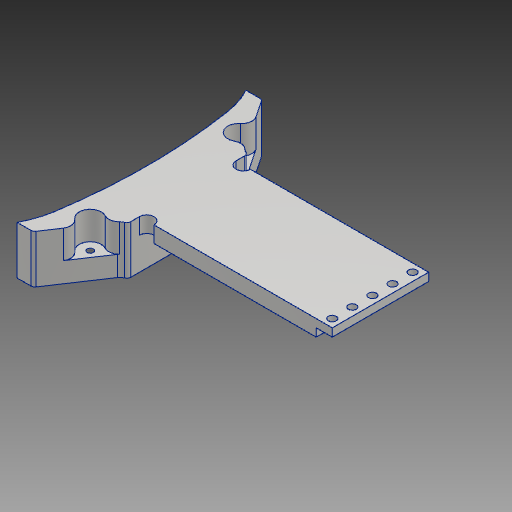
# Autodesk Inventor part: Kicker Sichel
Saved by Autodesk Inventor 2019.4 (Build 234330000, 330)
## iProperties
Part Number: Kicker Sichel
Material: Aluminium 6061
Document SubType Name: Modeling
Designer: rYan
Mass: 26.3222 g
Surface Area: 53.2988 cm^2
Volume: 9.74896 cm^3
Density: 2.7 g/cm^3
Appearance: Aluminium - flach
Author: rYan
Autodesk Inventor part; units mm, degrees
ref_plane "YZ Plane" through (0, 0, 0) normal (1, 0, 0) x (0, 1, 0)
ref_plane "XZ Plane" through (0, 0, 0) normal (0, 1, 0) x (-1, 0, 0)
ref_plane "XY Plane" through (0, 0, 0) normal (0, 0, 1) x (1, 0, 0)
sketch "Skizze1" plane through (0, 0, 0) normal (0, 0, 1) x (1, 0, 0)
  line L0 (3.6, 12) -> (48, 12)
  line L1 (48, 12) -> (48, -12)
  line L2 (48, -12) -> (3.6, -12)
  line L3 (-189.6, 0) -> (87.6, 0) projected
  line L4 (-1, 15) -> (-10, 28.5)
  line L5 (-1, -15) -> (-10, -28.5)
  line L6 (-10, -28.5) -> (-14, -28.5)
  line L7 (-10, 28.5) -> (-14, 28.5)
  arc A0 (-11.6616, 21.5053) -> (-14, 28.5) centre (-33.4005, 18.1259) ccw
  arc A1 (-14, -28.5) -> (-11.6616, -21.5053) centre (-33.4005, -18.1259) ccw
  arc A2 (-11.6616, -21.5053) -> (-11.6616, 21.5053) centre (-150, 0) ccw
  line L8 (-10, 28.5) -> (-10, -28.5) construction
  line L9 (0, 40.0382) -> (0, -40.0382) projected
  line L10 (-2, 12.5) -> (-2, -9.8115) construction
  arc A3 (0, 12) -> (3.6, 12) centre (1.8, 12) ccw
  arc A4 (3.6, -12) -> (0, -12) centre (1.8, -12) ccw
  line L11 (0, 12) -> (0, 15)
  line L12 (0, 15) -> (-1, 15)
  line L13 (0, -12) -> (0, -15)
  line L14 (0, -15) -> (-1, -15)
  point P0 (0, 0)
  dimension "d2" = 24
  dimension "d51" = 22
  dimension "d52" = 140
  dimension "d54" = 4
  dimension "d55" = 57
  dimension "d59" = 8
  dimension "d60" = 2
  dimension "d64" = 0
  dimension "d73" = 1.8
  dimension "d75" = 48
  dimension "d76" = 30
  dimension "d77" = 1
  constraints: 26 end point, 10 point on circle, 7 point on line, 5 centre point, 4 perpendicular, 3 horizontal, 3 tangent, 3 vertical, 1 parallel, 7 other
  measures "d2" distance of L0.end L1.end
  measures "d51" radius of A0
  measures "d52" radius of A2
  measures "d54" distance from line of L7.end L8
  measures "d55" distance between parallel lines of L6 L7
  measures "d59" distance between parallel lines of L10 L8
  measures "d60" distance between parallel lines of L9 L10
  measures "d64" distance from line of L8 L4.end
  measures "d73" radius of A3
  measures "d75" distance between parallel lines of L1 L9
  measures "d76" distance between parallel lines of L14 L12
  measures "d77" distance of L11.end L4.start
extrude "Extrusion1" add sketch "Skizze1" along normal blind 12
sketch "Skizze8" plane through (0, 0, 12) normal (0, 0, 1) x (1, 0, 0)
  line L0 (-189.6, 0) -> (87.6, 0) projected
  arc A0 (-11.6616, -21.5053) -> (-11.6616, 21.5053) centre (-150, 0) ccw projected
  line L1 (-1, 15) -> (-10, 28.5) projected
  line L2 (-11.2277, 18.5) -> (-3.3333, 18.5) construction
  point P0 (0, 0)
  point P1 (-5.7805, 18.5)
  point P2 (-5.7805, -18.5)
  point P3 (-7.2805, 18.5)
  dimension "d65" = 18.5
  dimension "d80" = 1.5
  constraints: 2 end point, 2 point on line, 1 horizontal, 1 midpoint, 1 point on circle, 1 symmetric about line
  measures "d65" distance between parallel lines of L0 L2
  measures "d80" distance of point (-7.281, 18.5) point (-5.781, 18.5)
hole "Bohrung4" at (-5.7805, 18.5, 12) at (-5.7805, -18.5, 12) direction (0, 0, -1) diameter 1.567 end through all counterbore diameter 5.5 counterbore depth 7 thread size "M2x0.4" class "6H" standard "ISO Metric profile"
sketch "Skizze2" plane through (0, 0, 0) normal (0, 0, -1) x (-1, 0, 0)
  line L0 (-48, -12) -> (-3.6, -12) projected
  line L1 (-48, 12) -> (-48, -12) projected
  line L2 (-48, 12) -> (-3.6, 12) projected
  line L3 (0, -12) -> (-48, -12)
  line L4 (-48, -12) -> (-48, 12)
  line L5 (-48, 12) -> (0, 12)
  line L6 (-3.6, 12) -> (-48, 12) projected
  line L7 (0, 12) -> (0, -12)
  point P0 (0, 0)
  point P1 (0, -12.5)
  point P2 (0, 12.5)
  point P3 (-3.6, -12)
  constraints: 8 end point, 2 horizontal, 1 midpoint, 1 parallel, 1 perpendicular, 1 vertical, 4 other
extrude "Extrusion2" cut sketch "Skizze2" against normal blind 8
sketch "Skizze3" plane through (0, 0, 8) normal (0, 0, -1) x (-1, 0, 0)
  line L0 (-3.6, -12) -> (-48, -12) projected
  line L1 (-48, -12) -> (-48, 12) projected
  line L2 (-48, 12) -> (-3.6, 12) projected
  line L3 (-48, -12) -> (-44, -12)
  line L4 (-44, -12) -> (-44, 12)
  line L5 (-44, 12) -> (-48, 12)
  line L6 (-48, 12) -> (-48, -12)
  point P0 (0, 0)
  point P1 (0, -12.5)
  point P2 (0, 12.5)
  point P3 (10, -12.5)
  point P4 (-3.6, 12)
  dimension "d9" = 4
  constraints: 8 end point, 2 parallel, 1 horizontal, 1 perpendicular, 3 other
  measures "d9" distance between parallel lines of L1 L4
extrude "Extrusion3" cut sketch "Skizze3" against normal blind 2
sketch "Skizze4" plane through (0, 0, 12) normal (0, 0, 1) x (1, 0, 0)
  line L0 (48, -12) -> (48, 12) projected
  line L1 (-26.4, 0) -> (60.4, 0) projected
  point P0 (0, 0)
  point P1 (46, 0)
  dimension "d12" = 2
  constraints: 1 point on line
  measures "d12" distance from line of L0 point (46, 0)
hole "Bohrung1" at (46, 0, 12) direction (0, 0, -1) diameter 2 end through all
pattern_linear "Rechteckige Anordnung1" count 5 spacing 5 along (0, 1, 0) of "Bohrung1" first direction both ways yes
sketch "Skizze7" plane through (0, 0, 12) normal (0, 0, 1) x (1, 0, 0)
  line L0 (-1, 15) -> (-3.061, 18.0915) projected
  line L1 (-10, 28.5) -> (-14, 28.5) projected
  arc A0 (-11.6616, 21.5053) -> (-14, 28.5) centre (-33.4005, 18.1259) ccw projected
  arc A1 (-11.6616, -21.5053) -> (-11.6616, 21.5053) centre (-150, 0) ccw projected
  arc A2 (-14, -28.5) -> (-11.6616, -21.5053) centre (-33.4005, -18.1259) ccw projected
  line L2 (-14, -28.5) -> (-10, -28.5) projected
  line L3 (-10, -28.5) -> (-5.1116, -21.1674) projected
  line L4 (3.6, -12) -> (48, -12) projected
  line L5 (48, -12) -> (48, 12) projected
  line L6 (48, 12) -> (3.6, 12) projected
  line L7 (-3, 28.5) -> (-14, 28.5)
  line L8 (-14, 28.5) -> (-14, -28.5)
  line L9 (-14, -28.5) -> (-3, -28.5)
  line L10 (-3, -28.5) -> (-3, 28.5)
  line L11 (-10, 28.5) -> (-14, 28.5) projected
  line L12 (-14, -28.5) -> (-10, -28.5) projected
  line L13 (0, 12) -> (0, 15) projected
  line L14 (0, 15) -> (-1, 15) projected
  line L15 (-1, -15) -> (0, -15) projected
  line L16 (0, -15) -> (0, -12) projected
  arc A3 (3.6, -12) -> (0, -12) centre (1.8, -12) ccw projected
  arc A4 (0, 12) -> (3.6, 12) centre (1.8, 12) ccw projected
  arc A5 (-5.1116, 21.1674) -> (-3.061, 18.0915) centre (-5.7805, 18.5) ccw projected
  arc A6 (-3.061, -18.0915) -> (-5.1116, -21.1674) centre (-5.7805, -18.5) ccw projected
  line L17 (-1, -15) -> (0, -15) projected
  line L18 (0, 15) -> (-1, 15) projected
  line L19 (-194.4, 0) -> (88.4, 0) projected
  line L20 (-1, 15) -> (-2, 15)
  line L21 (0, -15) -> (-1, -15) projected
  line L22 (-2, -15) -> (-1, -15)
  line L23 (-5.1116, 21.1674) -> (-10, 28.5) projected
  line L24 (-3.061, -18.0915) -> (-1, -15) projected
  point P0 (0.6841, -13.8749)
  point P1 (0, 0)
  point P2 (-3, -14)
  point P3 (-3, 14)
  dimension "d86" = 3
  constraints: 12 end point, 5 point on line, 4 equal length, 2 collinear, 1 horizontal, 1 perpendicular
  measures "d86" distance from line of point (0, 0) L10
extrude "Extrusion4" [suppressed]
fillet "Rundung1" radius 2 2 edges at (-1, -15, 6) (-1, 15, 6)
fillet "Rundung2" radius 1 4 edges at (-10, -28.5, 6) (-10, 28.5, 6) (0, -15.0012, 6) (0, 15.0012, 6)
fillet "Rundung3" radius 2.5 4 edges at (-5.1116, -21.1674, 8.5) (-3.061, -18.0915, 8.5) (-5.1116, 21.1674, 8.5) (-3.061, 18.0915, 8.5)
chamfer "Fase1" [suppressed]
sketch "Skizze9" plane through (0, 0, 7) normal (0, 0, 1) x (1, 0, 0)
  arc A0 (-10.4764, 20.7604) -> (-7.2043, 16.343) centre (-8.9101, 18.5) ccw projected
  line L0 (-12.7002, 28.0952) -> (-9.8914, 24.3034) projected
  arc A1 (-12.7002, 28.0952) -> (-13.5037, 28.5) centre (-13.5037, 27.5) ccw projected
  line L1 (-18, 28.5) -> (-13.5037, 28.5) projected
  arc A2 (-15.6616, 21.5053) -> (-18, 28.5) centre (-37.4005, 18.1259) ccw projected
  arc A3 (-15.6616, -21.5053) -> (-15.6616, 21.5053) centre (-154, 0) ccw projected
  arc A4 (-18, -28.5) -> (-15.6616, -21.5053) centre (-37.4005, -18.1259) ccw projected
  line L2 (-13.5037, -28.5) -> (-18, -28.5) projected
  arc A5 (-13.5037, -28.5) -> (-12.7002, -28.0952) centre (-13.5037, -27.5) ccw projected
  line L3 (-9.8914, -24.3034) -> (-12.7002, -28.0952) projected
  arc A6 (-7.2043, -16.343) -> (-10.4764, -20.7604) centre (-8.9101, -18.5) ccw projected
  line L4 (-3, 12) -> (-4, 12)
  line L5 (-4, 12) -> (-4, -12)
  line L6 (-4, -12) -> (-3, -12)
  line L7 (-3, -12) -> (-3, 12)
  line L8 (-194.4, 0) -> (88.4, 0) projected
  line L9 (-3, 15.2723) -> (-3, -15.2723) projected
  arc A7 (-3, -15.2723) -> (-3.5997, -15.8095) centre (-1.9925, -17) ccw projected
  arc A8 (-3.5997, 15.8095) -> (-3, 15.2723) centre (-1.9925, 17) ccw projected
  arc A9 (-3.6446, 15.8702) -> (-7.2043, 16.343) centre (-5.6535, 14.3821) ccw projected
  arc A10 (-10.4764, 20.7604) -> (-9.8914, 24.3034) centre (-11.9003, 22.8153) ccw projected
  arc A11 (-9.8914, -24.3034) -> (-10.4764, -20.7604) centre (-11.9003, -22.8153) ccw projected
  arc A12 (-7.2043, -16.343) -> (-3.6446, -15.8702) centre (-5.6535, -14.3821) ccw projected
  line L10 (-3.5997, -15.8095) -> (-3.6446, -15.8702) projected
  line L11 (-3.6446, 15.8702) -> (-3.5997, 15.8095) projected
  point P0 (0, 0)
  dimension "d88" = 1
  dimension "d89" = 24
  constraints: 8 end point, 2 parallel, 1 horizontal, 1 perpendicular, 1 other
  measures "d88" distance of L4.start L4.end
  measures "d89" distance of L4.end L5.end
extrude "Extrusion5" [suppressed]
sketch "Skizze10" plane through (0, 0, 7) normal (0, 0, 1) x (1, 0, 0)
  arc A0 (-10.4764, 20.7604) -> (-7.2043, 16.343) centre (-8.9101, 18.5) ccw projected
  arc A1 (-12.7002, 28.0952) -> (-13.5037, 28.5) centre (-13.5037, 27.5) ccw projected
  line L0 (-18, 28.5) -> (-13.5037, 28.5) projected
  arc A2 (-15.6616, 21.5053) -> (-18, 28.5) centre (-37.4005, 18.1259) ccw projected
  arc A3 (-15.6616, -21.5053) -> (-15.6616, 21.5053) centre (-154, 0) ccw projected
  arc A4 (-18, -28.5) -> (-15.6616, -21.5053) centre (-37.4005, -18.1259) ccw projected
  line L1 (-13.5037, -28.5) -> (-18, -28.5) projected
  arc A5 (-13.5037, -28.5) -> (-12.7002, -28.0952) centre (-13.5037, -27.5) ccw projected
  line L2 (-9.8914, -24.3034) -> (-12.7002, -28.0952) projected
  arc A6 (-7.2043, -16.343) -> (-10.4764, -20.7604) centre (-8.9101, -18.5) ccw projected
  line L3 (-4, 12) -> (-5, 12)
  line L4 (-5, 12) -> (-5, -12)
  line L5 (-5, -12) -> (-4, -12)
  line L6 (-4, -12) -> (-4, 12)
  line L7 (-3, 15.2723) -> (-3, -15.2723) projected
  line L8 (-12.7002, 28.0952) -> (-9.8914, 24.3034) projected
  arc A7 (-3.5997, 15.8095) -> (-3, 15.2723) centre (-1.9925, 17) ccw projected
  arc A8 (-3, -15.2723) -> (-3.5997, -15.8095) centre (-1.9925, -17) ccw projected
  line L9 (-3.6446, 15.8702) -> (-3.5997, 15.8095) projected
  arc A9 (-3.6446, 15.8702) -> (-7.2043, 16.343) centre (-5.6535, 14.3821) ccw projected
  arc A10 (-10.4764, 20.7604) -> (-9.8914, 24.3034) centre (-11.9003, 22.8153) ccw projected
  arc A11 (-9.8914, -24.3034) -> (-10.4764, -20.7604) centre (-11.9003, -22.8153) ccw projected
  arc A12 (-7.2043, -16.343) -> (-3.6446, -15.8702) centre (-5.6535, -14.3821) ccw projected
  line L10 (-3.5997, -15.8095) -> (-3.6446, -15.8702) projected
  point P0 (0, 0)
  dimension "d92" = 1
  constraints: 8 end point, 2 parallel, 1 horizontal, 1 perpendicular, 1 point on line
  measures "d92" distance of L3.start L3.end
extrude "Extrusion6" [suppressed]
fillet "Rundung4" [suppressed]
chamfer "Fase3" [suppressed]
